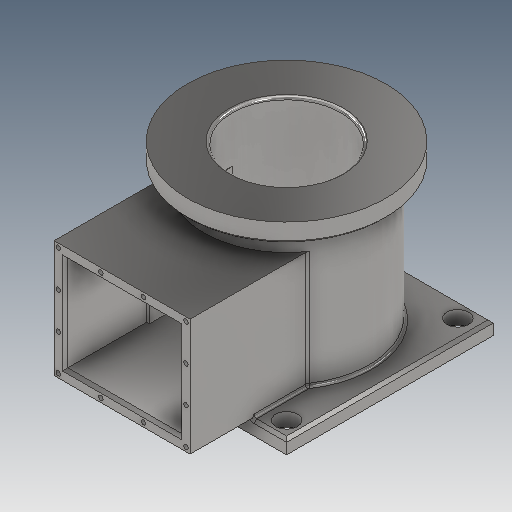
# Autodesk Inventor part: Ground base of robot
Saved by Autodesk Inventor 2020.3 (Build 243373010, 373A)
## iProperties
Created: 2021-04-17
Part Number: Ground base of robot
Material: Steel, Cast
Document SubType Name: Modeling
Designer: marti
Density: 7.85 g/cm^3
Appearance: Steel - Polished
Mass: 136890 g
Surface Area: 10903.6 cm^2
Volume: 17438.2 cm^3
Author: marti
Autodesk Inventor part; units mm, degrees
ref_plane "YZ Plane" through (0, 0, 0) normal (1, 0, 0) x (0, 1, 0)
ref_plane "XZ Plane" through (0, 0, 0) normal (0, 1, 0) x (-1, 0, 0)
sketch "Sketch1" plane through (0, 0, 0) normal (0, 1, 0) x (-1, 0, 0)
  circle A0 centre (0, 0) radius 182.5
  dimension "d0" = 365
  constraints: 1 centre point, 1 coincident
  measures "d0" diameter of A0
extrude "Extrusion1" add sketch "Sketch1" against normal blind 35
sketch "Sketch2" plane through (0, 0, 0) normal (0, 1, 0) x (1, 0, 0)
  circle A0 centre (0, 0) radius 100
  dimension "d3" = 200
  constraints: 1 centre point, 1 coincident
  measures "d3" diameter of A0
extrude "Extrusion2" cut sketch "Sketch2" against normal through all
sketch "Sketch3" plane through (0, -35, 0) normal (0, -1, 0) x (1, 0, 0)
  circle A0 centre (0, 0) radius 182.5 projected
  circle A1 centre (0, 0) radius 100 projected
  circle A2 centre (0, 0) radius 152.5
  dimension "d6" = 365
  dimension "d7" = 305
  constraints: 1 centre point, 1 coincident
  measures "d6" diameter of A0
  measures "d7" diameter of A2
extrude "Extrusion3" add sketch "Sketch3" along normal blind 250 contours A2
ref_plane "Work Plane1" through (0, 0, 152.5) normal (0, 0, 1) x (1, 0, 0)
sketch "Sketch4" plane through (0, 0, 152.5) normal (0, 0, 1) x (1, 0, 0)
  line L0 (-125, -70) -> (125, -70)
  line L1 (-152.5, -285) -> (152.5, -285) projected
  line L2 (152.5, -35) -> (-152.5, -35) projected
  line L3 (-152.5, -35) -> (-152.5, -285) projected
  line L4 (152.5, -35) -> (152.5, -285) projected
  line L5 (-125, -70) -> (-125, -285)
  line L6 (-152.5, -285) -> (152.5, -285) projected
  line L7 (125, -70) -> (125, -285)
  point P0 (0, 0)
  point P1 (0, -70)
  point P2 (0, -285)
  point P3 (0, -285)
  dimension "d11" = 215
  dimension "d12" = 250
  constraints: 6 end point, 2 midpoint, 2 point on line, 1 coincident, 1 horizontal, 1 perpendicular, 1 vertical, 1 vertical alignment
  measures "d11" distance between parallel lines of L1 L0
  measures "d12" distance of L0.start L0.end
extrude "Extrusion4" add sketch "Sketch4" against normal up to next contours L0 L7 L1 L5
extrude "Extrusion5" add sketch "Sketch4" along normal blind 150 contours L0 L7 L1 L5
sketch "Sketch5" plane through (0, -285, 0) normal (0, -1, 0) x (1, 0, 0)
  line L0 (190, 190) -> (-190, 190)
  line L1 (-190, 190) -> (-190, -190)
  line L2 (-190, -190) -> (190, -190)
  line L3 (190, -190) -> (190, 190)
  point P0 (0, 0)
  dimension "d57" = 380
  dimension "d58" = 380
  constraints: 8 end point, 2 parallel, 1 horizontal, 1 perpendicular
  measures "d57" distance between parallel lines of L3 L1
  measures "d58" distance between parallel lines of L0 L2
extrude "Extrusion6" add sketch "Sketch5" along normal blind 25
sketch "Sketch7" plane through (0, 0, 302.5) normal (0, 0, 1) x (1, 0, 0)
  line L0 (-105, -90) -> (105, -90)
  line L1 (105, -90) -> (105, -265)
  line L2 (105, -265) -> (-105, -265)
  line L3 (-105, -265) -> (-105, -90)
  line L4 (125, -70) -> (-125, -70) projected
  line L5 (-125, -70) -> (-125, -285) projected
  line L6 (-125, -285) -> (125, -285) projected
  line L7 (125, -285) -> (125, -70) projected
  point P0 (0, 0)
  dimension "d19" = 20
  dimension "d20" = 20
  dimension "d21" = 20
  dimension "d22" = 20
  constraints: 8 end point, 2 parallel, 1 horizontal, 1 perpendicular
  measures "d19" distance between parallel lines of L4 L0
  measures "d20" distance between parallel lines of L5 L3
  measures "d21" distance between parallel lines of L6 L2
  measures "d22" distance between parallel lines of L7 L1
extrude "Extrusion7" cut sketch "Sketch7" against normal blind 150 contours L0 L1 L2 L3
sketch "Sketch8" plane through (0, 0, 152.5) normal (0, 0, 1) x (1, 0, 0)
  line L0 (-100, 0) -> (100, 0) projected
  line L1 (100, -285) -> (-100, -285) projected
  line L2 (-100, 0) -> (100, 0) projected
  line L3 (-100, 0) -> (-100, -285)
  line L4 (-100, 0) -> (-100, -285) projected
  line L5 (100, 0) -> (100, -285)
  line L6 (105, -90) -> (105, -265) projected
  line L7 (105, -265) -> (-105, -265) projected
  line L8 (105, -90) -> (105, -265) projected
  line L9 (-105, -90) -> (105, -90) projected
  line L10 (-105, -265) -> (-105, -90) projected
  point P0 (0, 0)
  point P1 (100, -90)
  point P2 (-100, -90)
  point P3 (-100, -265)
  point P4 (100, -265)
  constraints: 4 end point, 1 collinear, 1 parallel
extrude "Extrusion8" cut sketch "Sketch8" against normal up to surface contours L9 L5 L7 L3 round surface about axis through (0, 0, 0) along (0, -1, 0) radius 100 far side no
fillet "Fillet1" radius 15 1 edges at (-100, -285, 0)
chamfer "Chamfer1" distance 5 angle 45 4 edges at (-105, -177.5, 302.5) (0, -90, 302.5) (105, -177.5, 302.5) (0, -265, 302.5)
fillet "Fillet2" radius 10 2 edges at (125, -177.5, 87.357) (-125, -177.5, 87.357)
fillet "Fillet3" radius 2 1 edges at (-152.5, -35, 0)
chamfer "Chamfer2" distance 5 angle 45 1 edges at (182.5, -35, 0)
fillet "Fillet4" radius 5 1 edges at (-100, 0, 0)
fillet "Fillet5" radius 5 6 edges at (125.4324, -285, 87.5414) (125, -285, 140.2251) (-125.4324, -285, 87.5414) (-125, -285, 140.2251) (-44.3603, -285, -145.9055) (145.9055, -285, 44.3603)
chamfer "Chamfer3" distance 5 angle 45 7 edges at (190, -285, 0) (0, -285, -190) (-190, -285, 0) (-160, -285, 190) (-126.4645, -283.5355, 190) (160, -285, 190) (126.4645, -283.5355, 190)
sketch "Sketch9" plane through (0, -285, 0) normal (0, 1, 0) x (1, 0, 0)
  circle A0 centre (-160, -160) radius 20
  line L0 (-190, -190) -> (-130, -190) projected
  line L1 (-190, 190) -> (-190, -190) projected
  circle A1 centre (-160, 160) radius 20
  line L2 (190, 190) -> (-190, 190) projected
  circle A2 centre (155, 160) radius 20
  line L3 (185, 185) -> (185, -185) projected
  circle A3 centre (160, -160) radius 20
  line L4 (190, -190) -> (190, 190) projected
  line L5 (130, -190) -> (190, -190) projected
  point P0 (0, 0)
  dimension "d41" = 40
  dimension "d42" = 30
  dimension "d43" = 30
  dimension "d44" = 40
  dimension "d45" = 30
  dimension "d48" = 40
  dimension "d50" = 30
  dimension "d51" = 40
  dimension "d52" = 30
  dimension "d53" = 30
  constraints: 4 centre point, 1 horizontal alignment, 1 vertical alignment
  measures "d41" diameter of A0
  measures "d42" distance from line of A0.centre L0
  measures "d43" distance from line of L1 A0.centre
  measures "d44" diameter of A1
  measures "d45" distance from line of L2 A1.centre
  measures "d48" diameter of A2
  measures "d50" distance from line of L3 A2.centre
  measures "d51" diameter of A3
  measures "d52" distance from line of L4 A3.centre
  measures "d53" distance from line of L5 A3.centre
extrude "Extrusion9" cut sketch "Sketch9" against normal through all
sketch "Sketch10" plane through (0, 0, 302.5) normal (0, 0, 1) x (1, 0, 0)
  line L0 (125, -285) -> (125, -70) projected
  line L1 (-125, -70) -> (-125, -285) projected
  line L2 (110, -85) -> (-110, -85) projected
  line L3 (125, -70) -> (-125, -70) projected
  line L4 (-110, -85) -> (-110, -270) projected
  line L5 (-125, -285) -> (125, -285) projected
  line L6 (-200.4459, -177.5) -> (246.7642, -177.5)
  line L7 (0, -70) -> (0, -285)
  point P0 (0, 0)
  point P1 (-117.5, -77.5)
  point P2 (-39.1667, -77.5)
  point P3 (39.1667, -77.5)
  point P4 (117.5, -77.5)
  point P5 (-117.5, -144.1667)
  point P6 (-117.5, -210.8333)
  point P7 (-117.5, -277.5)
  point P8 (-39.1667, -277.5)
  point P9 (39.1667, -277.5)
  point P10 (117.5, -277.5)
  point P11 (117.5, -144.1667)
  point P12 (117.5, -210.8333)
  dimension "d59" = 250
  dimension "d60" = 15
  dimension "d61" = 15
  dimension "d62" = 7.5
  dimension "d63" = 7.5
  dimension "d66" = 78.3333
  dimension "d71" = 215
  dimension "d74" = 66.6667
  dimension "d79" = 107.5
  constraints: 5 symmetric about line, 4 end point, 2 horizontal, 2 midpoint, 1 vertical, 6 other
  measures "d59" distance between parallel lines of L0 L1
  measures "d60" distance between parallel lines of L2 L3
  measures "d61" distance between parallel lines of L1 L4
  measures "d62" distance from line of L3 point (-117.5, -77.5)
  measures "d63" distance from line of L1 point (-117.5, -77.5)
  measures "d66" distance of point (-117.5, -77.5) point (-39.167, -77.5)
  measures "d71" distance between parallel lines of L5 L3
  measures "d74" distance of point (-117.5, -77.5) point (-117.5, -144.167)
  measures "d79" distance between parallel lines of L6 L3
hole "Hole1" at (-117.5, -77.5, 302.5) at (-39.1667, -77.5, 302.5) at (39.1667, -77.5, 302.5) at (117.5, -77.5, 302.5) at (-117.5, -144.1667, 302.5) at (-117.5, -210.8333, 302.5) at (-117.5, -277.5, 302.5) at (-39.1667, -277.5, 302.5) at (39.1667, -277.5, 302.5) at (117.5, -277.5, 302.5) at (117.5, -144.1667, 302.5) at (117.5, -210.8333, 302.5) direction (0, 0, -1) diameter 8.376 depth 27.3 tip angle 118 thread size "M10x1.5" class "6H" standard "ISO Metric profile"
equation "\"d62\" = 0.5 * d60"
equation "\"d63\" = 0.5 * d61"
equation "\"d79\" = 0.5 * d71"
body "Solid1"
